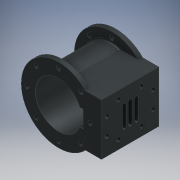
# Autodesk Inventor part: cylinder
Saved by Autodesk Inventor 2017 (Build 210142000, 142)
## iProperties
Created: 2018-11-18
Part Number: cylinder
Material: Iron, Cast
Document SubType Name: Modeling
Designer: Arman Grewal
Density: 7.15 g/cm^3
Appearance: Iron Gray
Author: Arman Grewal
Autodesk Inventor part; units mm, degrees
ref_plane "YZ Plane" through (0, 0, 0) normal (1, 0, 0) x (0, 1, 0)
ref_plane "XY Plane" through (0, 0, 0) normal (0, 0, 1) x (1, 0, 0)
sketch "Sketch1" plane through (0, 0, 0) normal (0, 1, 0) x (-1, 0, 0)
  circle A0 centre (0, 0) radius 16
  arc A1 (-6.0828, -18) -> (-6.0828, 18) centre (0, 0) ccw
  line L0 (-30, 0) -> (-30, -18)
  line L1 (-30, -18) -> (-30, 18)
  line L2 (-30, 18) -> (-6.0828, 18)
  line L3 (-30, -18) -> (-6.0828, -18)
  dimension "d0" = 32
  dimension "d1" = 36
  dimension "d2" = 19
  dimension "d3" = 18
  dimension "d4" = 30
  dimension "d5" = 18
  dimension "d6" = 30
  dimension "d7" = 18
  constraints: 8 end point, 2 centre point, 2 coincident, 2 point on circle, 1 horizontal, 1 parallel, 1 point on line, 1 vertical
  measures "d0" diameter of A0
  measures "d1" distance of L0.end L1.end
  measures "d2" radius of A1
  measures "d3" distance from line of point (0, 0) L2
  measures "d4" distance from line of point (0, 0) L1
  measures "d5" distance from line of point (0, 0) L2
  measures "d6" distance from line of point (0, 0) L1
  measures "d7" distance from line of L0.start L2
extrude "Extrusion1" add sketch "Sketch1" along normal blind 40
sketch "Sketch2" plane through (0, 40, 0) normal (0, 1, 0) x (1, 0, 0)
  arc A0 (18.7617, 18) -> (18.7617, -18) centre (0, 0) ccw
  arc A1 (6.0828, 18) -> (6.0828, -18) centre (0, 0) ccw construction
  circle A2 centre (0, 0) radius 22 construction
  circle A3 centre (-22, 0) radius 1.5
  circle A4 centre (-15.5563, -15.5563) radius 1.5
  circle A5 centre (0, -22) radius 1.5
  circle A6 centre (15.5563, -15.5563) radius 1.5
  circle A7 centre (22, 0) radius 1.5
  circle A8 centre (15.5563, 15.5563) radius 1.5
  circle A9 centre (0, 22) radius 1.5
  circle A10 centre (-15.5563, 15.5563) radius 1.5
  arc A11 (18.7617, 18) -> (18.7617, -18) centre (0, 0) ccw
  arc A12 (6.0828, 18) -> (6.0828, -18) centre (0, 0) ccw
  line L0 (6.0828, -18) -> (18.7617, -18)
  line L1 (6.0828, 18) -> (18.7617, 18)
  dimension "d12" = 44
  dimension "d13" = 3
  dimension "d14" = 360
  dimension "d15" = 26
  dimension "d16" = 19
  dimension "d17" = 36
  dimension "d18" = 18
  dimension "d19" = 18
  dimension "d20" = 2.4436
  dimension "d21" = 22
  constraints: 12 centre point, 8 point on circle, 4 coincident, 4 end point, 2 concentric, 1 horizontal, 1 horizontal alignment, 1 parallel, 19 other
  measures "d13" diameter of A3
  measures "d15" radius of A0
  measures "d16" radius of A12
  measures "d17" distance between parallel lines of L1 L0
  measures "d18" distance from line of point (0, 0) L1
  measures "d19" distance from line of A7.centre L1
  measures "d20" distance from line of A8.centre L1
  measures "d21" distance of point (0, 0) A7.centre
extrude "Extrusion2" add sketch "Sketch2" against normal blind 3 contours L1 A12 L0 A0
sketch "Sketch3" plane through (0, 40, 0) normal (0, 1, 0) x (1, 0, 0)
  arc A0 (18.7617, 18) -> (18.7617, -18) centre (0, 0) ccw
  arc A1 (6.0828, 18) -> (6.0828, -18) centre (0, 0) ccw construction
  circle A2 centre (0, 0) radius 22 construction
  circle A3 centre (-22, 0) radius 1.5
  circle A4 centre (-15.5563, -15.5563) radius 1.5
  circle A5 centre (0, -22) radius 1.5
  circle A6 centre (15.5563, -15.5563) radius 1.5
  circle A7 centre (22, 0) radius 1.5
  circle A8 centre (15.5563, 15.5563) radius 1.5
  circle A9 centre (0, 22) radius 1.5
  circle A10 centre (-15.5563, 15.5563) radius 1.5
  arc A11 (18.7617, 18) -> (18.7617, -18) centre (0, 0) ccw
  arc A12 (6.0828, 18) -> (6.0828, -18) centre (0, 0) ccw
  line L0 (6.0828, -18) -> (18.7617, -18)
  line L1 (6.0828, 18) -> (18.7617, 18)
  dimension "d26" = 44
  dimension "d27" = 3
  dimension "d28" = 360
  dimension "d29" = 26
  dimension "d30" = 19
  dimension "d31" = 36
  dimension "d32" = 18
  dimension "d33" = 18
  dimension "d34" = 2.4436
  dimension "d35" = 22
  constraints: 12 centre point, 8 point on circle, 4 coincident, 4 end point, 2 concentric, 1 horizontal, 1 horizontal alignment, 1 parallel, 19 other
  measures "d27" diameter of A3
  measures "d29" radius of A0
  measures "d30" radius of A12
  measures "d31" distance between parallel lines of L1 L0
  measures "d32" distance from line of point (0, 0) L1
  measures "d33" distance from line of A7.centre L1
  measures "d34" distance from line of A8.centre L1
  measures "d35" distance of point (0, 0) A7.centre
extrude "Extrusion3" cut sketch "Sketch3" against normal blind 5 contours A6 | A7 | A8
sketch "Sketch4" plane through (30, 0, 18) normal (1, 0, 0) x (0, 0, -1)
  line L0 (18, 0) -> (18, 40) construction
  line L1 (0, 40) -> (36, 40) construction
  line L2 (0, 0) -> (0, 37) construction
  line L3 (0, 20) -> (36, 20) construction
  line L4 (36, 0) -> (36, 37) construction
  line L5 (0, 20) -> (0, 28) construction
  line L6 (0, 28) -> (0, 12) construction
  line L7 (2, 0) -> (2, 40) construction
  line L8 (2, 28) -> (34, 28) construction
  line L9 (34, 0) -> (34, 40) construction
  line L10 (2, 12) -> (34, 12) construction
  line L11 (18, 0) -> (24, 0) construction
  line L12 (36, 0) -> (0, 0) construction
  line L13 (24, 0) -> (12, 0) construction
  line L14 (0, 20) -> (0, 36) construction
  line L15 (0, 36) -> (0, 4) construction
  line L16 (0, 4) -> (36, 4) construction
  line L17 (0, 36) -> (36, 36) construction
  line L18 (24, 0) -> (24, 40) construction
  line L19 (12, 0) -> (12, 40) construction
  line L20 (0, 36) -> (6, 36) construction
  line L21 (36, 36) -> (30, 36) construction
  line L22 (6, 40) -> (6, 0) construction
  line L23 (30, 40) -> (30, 0) construction
  circle A0 centre (6, 28) radius 1.5
  circle A1 centre (12, 36) radius 1.5
  circle A2 centre (24, 36) radius 1.5
  circle A3 centre (30, 28) radius 1.5
  circle A4 centre (30, 12) radius 1.5
  circle A5 centre (6, 12) radius 1.5
  circle A6 centre (12, 4) radius 1.5
  circle A7 centre (24, 4) radius 1.5
  line L24 (36, 0) -> (36, 40)
  line L25 (18, 17.25) -> (11.25, 17.25)
  line L26 (11.25, 17.25) -> (24.75, 17.25)
  line L27 (24.75, 14.75) -> (11.25, 14.75)
  line L28 (18, 23.25) -> (24.75, 23.25)
  line L29 (24.75, 25.75) -> (11.25, 25.75)
  line L30 (11.25, 23.25) -> (18, 23.25)
  arc A8 (11.25, 25.75) -> (11.25, 23.25) centre (11.25, 24.5) ccw
  arc A9 (24.75, 23.25) -> (24.75, 25.75) centre (24.75, 24.5) ccw
  arc A10 (11.25, 17.25) -> (11.25, 14.75) centre (11.25, 16) ccw
  arc A11 (24.75, 14.75) -> (24.75, 17.25) centre (24.75, 16) ccw
  line L31 (18, 18.75) -> (24.75, 18.75)
  line L32 (24.75, 18.75) -> (11.25, 18.75)
  line L33 (11.25, 21.75) -> (24.75, 21.75)
  arc A12 (11.25, 21.75) -> (11.25, 18.75) centre (11.25, 20.25) ccw
  arc A13 (24.75, 18.75) -> (24.75, 21.75) centre (24.75, 20.25) ccw
  dimension "d38" = 8
  dimension "d39" = 16
  dimension "d40" = 6
  dimension "d41" = 12
  dimension "d42" = 16
  dimension "d43" = 32
  dimension "d44" = 6
  dimension "d45" = 6
  dimension "d46" = 3
  dimension "d47" = 3
  dimension "d48" = 3
  dimension "d49" = 3
  dimension "d50" = 3
  dimension "d51" = 3
  dimension "d52" = 3
  dimension "d53" = 3
  dimension "d54" = 90
  dimension "d55" = 36
  dimension "d56" = 28
  dimension "d57" = 12
  dimension "d58" = 40
  dimension "d59" = 2
  dimension "d60" = 6
  dimension "d61" = 12
  dimension "d62" = 30
  dimension "d63" = 34
  dimension "d64" = 36
  dimension "d65" = 0
  dimension "d66" = 18
  dimension "d67" = 0
  dimension "d68" = 37
  dimension "d69" = 40
  dimension "d70" = 2
  dimension "d71" = 0
  dimension "d72" = 40
  dimension "d73" = 34
  dimension "d74" = 0
  dimension "d75" = 37
  dimension "d76" = 2.5
  dimension "d77" = 2.5
  dimension "d78" = 23.25
  dimension "d79" = 18.75
  dimension "d80" = 17.25
  dimension "d81" = 0
  dimension "d83" = 40
  dimension "d84" = 0
  dimension "d85" = 11.25
  dimension "d87" = 11.25
  dimension "d88" = 18
  dimension "d89" = 18
  dimension "d90" = 18
  dimension "d91" = 0
  dimension "d92" = 18
  dimension "d93" = 24.75
  dimension "d94" = 24.75
  dimension "d95" = 24.75
  dimension "d103" = 11.25
  constraints: 66 end point, 35 point on line, 14 centre point, 12 point on circle, 12 tangent, 9 parallel, 6 horizontal, 4 perpendicular, 3 vertical, 1 equal radius, 8 other
  measures "d38" distance of L3.start L6.start
  measures "d39" distance of L6.start L6.end
  measures "d40" distance of L11.start L13.start
  measures "d41" distance of L13.start L13.end
  measures "d42" distance of L3.start L17.start
  measures "d43" distance of L17.start L15.end
  measures "d44" distance of L17.start L20.end
  measures "d45" distance of L17.end L21.end
  measures "d46" diameter of A0
  measures "d47" diameter of A1
  measures "d48" diameter of A2
  measures "d49" diameter of A3
  measures "d50" diameter of A4
  measures "d51" diameter of A5
  measures "d52" diameter of A6
  measures "d53" diameter of A7
  measures "d54" angle of L4 L11
  measures "d55" distance between parallel lines of L12 L17
  measures "d56" distance between parallel lines of L8 L12
  measures "d57" distance between parallel lines of L10 L12
  measures "d59" distance between parallel lines of L9 L4
  measures "d60" distance between parallel lines of L4 L23
  measures "d61" distance between parallel lines of L4 L18
  measures "d62" distance between parallel lines of L4 L22
  measures "d63" distance between parallel lines of L7 L4
  measures "d64" distance between parallel lines of L4 L2
  measures "d65" distance from line of point (18, 0) L12
  measures "d66" distance from line of point (18, 0) L4
  measures "d67" distance from line of point (36, 40) L4
  measures "d68" distance from line of L4.end L12
  measures "d69" distance from line of L9.end L12
  measures "d70" distance from line of L10.end L4
  measures "d71" distance from line of L9.start L12
  measures "d72" distance from line of L7.end L12
  measures "d73" distance from line of L10.start L4
  measures "d74" distance from line of L7.start L12
  measures "d75" distance from line of L2.end L12
  measures "d76" distance of L26.end L27.start
  measures "d77" distance of L28.end L29.start
  measures "d78" distance between parallel lines of L12 L28
  measures "d79" distance between parallel lines of L31 L12
  measures "d80" distance between parallel lines of L12 L26
  measures "d81" distance between parallel lines of L24 L4
  measures "d83" distance from line of L24.end L12
  measures "d84" distance from line of L24.start L12
  measures "d85" distance from line of L29.start L4
  measures "d87" distance from line of L26.end L4
  measures "d88" distance from line of L30.end L4
  measures "d89" distance from line of L31.start L4
  measures "d90" distance from line of L25.start L4
  measures "d91" distance from line of point (18, 0) L12
  measures "d92" distance from line of point (18, 0) L4
  measures "d93" distance from line of L29.end L4
  measures "d94" distance from line of L33.start L4
  measures "d95" distance from line of L25.end L4
  measures "d103" distance from line of L33.end L4
extrude "Extrusion4" cut sketch "Sketch4" against normal blind 10
ref_plane "Work Plane1" through (0, 20, 0) normal (0, 1, 0) x (-1, 0, 0)
mirror "Mirror1" about plane through (0, 20, 0) normal (0, 1, 0) of "Extrusion2", "Extrusion3"
sketch "Sketch5" plane through (30, 0, -18) normal (0, 0, -1) x (-1, 0, 0)
  circle A0 centre (5, 20) radius 1.5
  circle A1 centre (5, 20) radius 2.5
  line L0 (0, 0) -> (0, 40) projected
  point P0 (30, 0)
  dimension "d99" = 3
  dimension "d100" = 5
  dimension "d101" = 32.0156
  dimension "d102" = 5
  constraints: 2 centre point, 1 coincident
  measures "d99" diameter of A0
  measures "d100" diameter of A1
  measures "d101" distance of point (30, 0) A0.centre
  measures "d102" distance from line of L0 A0.centre
extrude "Extrusion5" cut sketch "Sketch5" against normal blind 11.25 contours A0
sketch "Sketch6" plane through (30, 0, -18) normal (0, 0, -1) x (-1, 0, 0)
  circle A0 centre (5, 20) radius 2.5
  line L0 (0, 0) -> (0, 40) projected
  point P0 (30, 0)
  dimension "d107" = 5
  dimension "d108" = 32.0156
  dimension "d109" = 5
  constraints: 1 centre point
  measures "d107" diameter of A0
  measures "d108" distance of point (30, 0) A0.centre
  measures "d109" distance from line of L0 A0.centre
extrude "Extrusion6" cut sketch "Sketch6" against normal blind 6
thread "Thread1" size "M5x0.8" class "6H" standard "ANSI Metric M Profile" full length
fillet "Fillet1" radius 1 2 edges at (-19, 37, 0) (-19, 3, 0)
sketch "Sketch10" plane through (0, 0, 0) normal (0, 0, 1) x (1, 0, 0)
  line L0 (-25.8287, 0.0788) -> (18.9329, 0.0788)
  line L1 (30.1713, 14.7288) -> (20.1713, 14.7288)
  line L2 (17.7727, 2.9788) -> (6.4163, 2.9788)
  line L3 (30.0713, 13.4788) -> (20.1713, 13.4788)
  line L4 (20.1713, 17.2288) -> (20.1713, 14.7288)
  line L5 (16, -0.0212) -> (-15.8287, -0.0212)
  line L6 (16, -0.0212) -> (17, -0.0212)
  line L7 (18.7941, -0.0212) -> (-25.7287, -0.0212)
  line L8 (16, -0.0212) -> (15, -0.0212)
  line L9 (20.1713, 17.2288) -> (15, 2.0181)
  line L10 (15, 2.0181) -> (15, -0.0212)
  line L11 (21.2418, 13.1454) -> (21.7519, 14.7288)
  line L12 (17, -0.0212) -> (21.2418, 13.1454)
  line L13 (30.1713, 17.2288) -> (20.1713, 17.2288)
  line L14 (20.1713, 17.2288) -> (20.1713, 14.7288)
  line L15 (21.7519, 14.7288) -> (20.1713, 14.7288)
  line L16 (16.1583, 0.5188) -> (16.1583, 39.9705)
  line L17 (16.1583, 20.2446) -> (18.7941, 20.2446)
  line L18 (20.1713, 23.2605) -> (20.1713, 25.7605)
  line L19 (20.1713, 23.2605) -> (15, 38.4712)
  line L20 (17, 40.5105) -> (21.2418, 27.3439)
  line L21 (21.2418, 27.3439) -> (21.7519, 25.7605)
  line L22 (21.7519, 25.7605) -> (20.1713, 25.7605)
  line L23 (15, 38.4712) -> (15, 40.5105)
  line L24 (16, 40.5105) -> (15, 40.5105)
  line L25 (16, 40.5105) -> (17, 40.5105)
  line L26 (23.5, 0) -> (20.5, 0) construction
  line L27 (16, 0) -> (-16, 0) construction
  line L28 (20.5, 0) -> (16, 0) construction
  point P0 (-1.657, -0.3388)
  point P1 (16.1583, 0.5188)
  dimension "d194" = 1
  dimension "d195" = 1
  dimension "d199" = 1
  dimension "d223" = 1
  dimension "d226" = 72.143
  dimension "d227" = 71.223
  dimension "d228" = 72.143
  dimension "d229" = 17.2288
  dimension "d230" = 14.7288
  dimension "d231" = 13.4788
  dimension "d232" = 20.2447
  dimension "d233" = 0.0212
  dimension "d234" = 2.9788
  dimension "d235" = 0.0788
  dimension "d236" = 4.013
  dimension "d237" = 5.1713
  dimension "d238" = 27.3439
  dimension "d239" = 0.3388
  dimension "d240" = 5.3975
  dimension "d241" = 8.0137
  dimension "d242" = 4.1524
  dimension "d243" = 1.1212
  dimension "d244" = 10.5584
  dimension "d245" = 4.5067
  dimension "d246" = 10.7212
  dimension "d247" = 10.7734
  dimension "d248" = 21.5827
  dimension "d249" = 30.2844
  dimension "d250" = 43.676
  dimension "d251" = 53.099
  dimension "d252" = 53.1636
  constraints: 48 end point, 8 symmetric about line, 6 parallel, 3 horizontal, 3 vertical, 2 collinear, 1 point on line, 12 other
  measures "d194" distance of L6.start L12.start
  measures "d195" distance of L6.start L10.end
  measures "d199" distance of point (16.158, 39.971) L20.start
  measures "d223" horizontal distance of L27.start L10.end
  measures "d226" angle of L26 L12
  measures "d227" angle of L26 L9
  measures "d228" angle to the sketch x axis of L21
  measures "d229" distance between parallel lines of L26 L13
  measures "d230" distance between parallel lines of L27 L15
  measures "d231" distance between parallel lines of L26 L3
  measures "d232" distance between parallel lines of L26 L17
  measures "d233" distance between parallel lines of L26 L6
  measures "d234" distance between parallel lines of L26 L2
  measures "d235" distance between parallel lines of L26 L0
  measures "d237" distance between parallel lines of L4 L10
  measures "d238" distance from line of L21.start L26
  measures "d239" distance from line of point (-1.657, -0.339) L26
  measures "d240" distance from line of L13.start L21
  measures "d241" distance from line of L1.start L11
  measures "d242" distance from line of L3.start L21
  measures "d243" distance from line of L3.end L11
  measures "d244" distance from line of L0.end L21
  measures "d245" distance from line of L17.end L21
  measures "d246" distance from line of point (18.794, -0.021) L21
  measures "d247" distance from line of L2.start L21
  measures "d248" distance from line of L2.end L21
  measures "d249" distance from line of point (-1.657, -0.339) L21
  measures "d250" distance from line of point (-15.829, -0.021) L21
  measures "d251" distance from line of point (-25.729, -0.021) L21
  measures "d252" distance from line of L0.start L21
extrude "Extrusion9" cut sketch "Sketch10" along normal mid plane 12
fillet "Fillet2" radius 0.1 75 edges at (-2.8284, 0, 15.748) (-2.8284, 0, -15.748) (-26, 0, 0) (-17.0563, 0, -15.5563) (-23.5, 0, 0) (-23.5, 3, 0) (-17.0563, 3, 15.5563) (-17.0563, 0, 15.5563) (-1.5, 3, 22) (-1.5, 0, 22) (14.0563, 0, 15.5563) (14.0563, 5, 15.5563) (20.5, 0, 0) (20.5, 5, 0) (14.0563, 0, -15.5563) (14.0563, 5, -15.5563) (30, 0, 0) (24.3808, 0, 18) (24.3808, 0, -18) (17.0068, 0, 0) (16.0034, 0, -6) (16.0034, 0, 6) (19.3794, 7.3644, 6) (19.3794, 7.3644, -6) (30, 20, -18) (30, 20, 18) (30, 40, 0) (30, 36, 7.5) (30, 36, -4.5) (30, 28, -10.5) (30, 12, -10.5) (30, 4, -4.5) (30, 4, 7.5) (30, 12, 13.5) (30, 28, 13.5) (30, 16, -8) (30, 14.75, 0) (30, 16, 8) (30, 17.25, 0) (30, 20.25, -8.25) (30, 18.75, 0) (30, 20.25, 8.25) (30, 21.75, 0) (30, 24.5, -8) (30, 23.25, 0) (30, 24.5, 8) (30, 25.75, 0) (27.5, 20, -18) (-26, 40, 0) (-26, 37, 0) (24.3808, 40, -18) (7.1809, 36.7842, -18) (13.7397, 37, -18) (7.1808, 3.2158, -18) (13.7397, 3, -18) (6.0828, 20, -18) (7.1809, 36.7842, 18) (13.7397, 37, 18) (7.1808, 3.2158, 18) (13.7397, 3, 18) (6.0828, 20, 18) (-2.8284, 40, 15.748) (-2.8284, 40, -15.748) (14.0563, 35, 15.5563) (14.0563, 40, 15.5563) (-1.5, 40, 22) (-1.5, 37, 22) (-17.0563, 40, 15.5563) (-17.0563, 37, 15.5563) (-23.5, 37, 0) (-23.5, 40, 0) (-17.0563, 40, -15.5563) (-1.5, 40, -22) (-1.5, 37, -22) (14.0563, 40, -15.5563)
fillet "Fillet3" radius 0.1 11 edges at (14.0563, 35, -15.5563) (20.5, 40, 0) (20.5, 35, 0) (29.9707, 39.9707, 17.9707) (24.3308, 40, 18) (18.6922, 40, 18) (17.1645, 40, 0) (19.4582, 32.8802, 6) (16.0822, 40, 6) (16.0822, 40, -6) (19.4582, 32.8802, -6)
body "Solid1"
